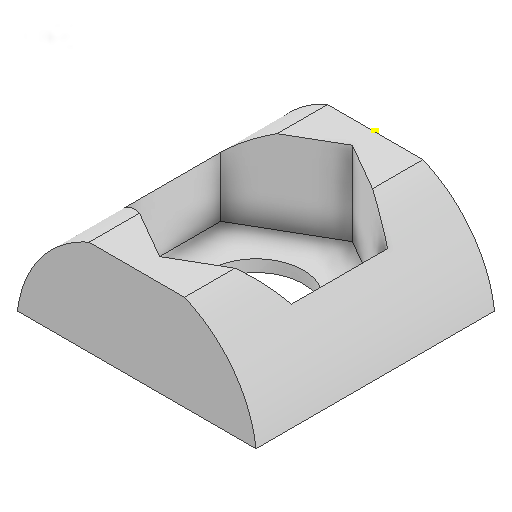
# Autodesk Inventor part: RailNut
Saved by Autodesk Inventor 2025.1 (Build 291241000, 241)
## iProperties
Created: 2025-03-12
Part Number: RailNut
Material: Generic
Document SubType Name: Modeling
Designer: rolan
Density: 1 g/cm^3
Appearance: Default
Author: rolan
Autodesk Inventor part; units mm, degrees
ref_plane "YZ Plane" through (0, 0, 0) normal (1, 0, 0) x (0, 1, 0)
ref_plane "XZ Plane" through (0, 0, 0) normal (0, 1, 0) x (-1, 0, 0)
ref_plane "XY Plane" through (0, 0, 0) normal (0, 0, 1) x (1, 0, 0)
sketch "Sketch1" plane through (0, 0, 0) normal (0, 0, 1) x (1, 0, 0)
  line L0 (-5, 0) -> (5, 0)
  line L1 (0, 0) -> (0, 4) construction
  line L2 (-2, 4) -> (2, 4)
  arc A0 (-2, 4) -> (-5, 0) centre (-0.0359, -0.5981) ccw
  arc A1 (5, 0) -> (2, 4) centre (0.0359, -0.5981) ccw
  dimension "d0" = 10
  dimension "d1" = 4
  dimension "d2" = 4
  dimension "d3" = 5
  dimension "d4" = 5
  constraints: 6 end point, 4 point on circle, 2 centre point, 2 horizontal, 2 midpoint, 1 vertical
  measures "d0" distance of L0.start L0.end
  measures "d1" distance of L1.start L1.end
  measures "d2" distance of L2.start L2.end
  measures "d3" radius of A0
  measures "d4" radius of A1
extrude "Extrusion1" add sketch "Sketch1" along normal blind 10
sketch "Sketch2" plane through (-2, 4, 0) normal (0, 1, 0) x (1, 0, 0)
  circle A0 centre (2, -5) radius 1.975
  line L0 (4, 0) -> (0, 0) projected
  line L1 (0, 0) -> (0, -10) projected
  point P0 (2, 0)
  point P1 (2, 0)
  dimension "d7" = 3.95
  dimension "d8" = 5
  dimension "d9" = 2
  constraints: 1 centre point, 1 midpoint
  measures "d7" diameter of A0
  measures "d8" distance of point (2, 0) A0.centre
  measures "d9" distance from line of L1 A0.centre
extrude "Extrusion2" cut sketch "Sketch2" against normal blind 10
sketch "Sketch3" plane through (-2, 4, 0) normal (0, 1, 0) x (1, 0, 0)
  point P0 (2, 0)
sketch "Sketch5" plane through (-2, 4, 0) normal (0, 1, 0) x (1, 0, 0)
  circle A0 centre (2, -5) radius 1.975 projected
  line L0 (2, -0.9585) -> (5.5, -2.9793)
  line L1 (5.5, -2.9793) -> (5.5, -7.0207)
  line L2 (5.5, -7.0207) -> (2, -9.0415)
  line L3 (2, -9.0415) -> (-1.5, -7.0207)
  line L4 (-1.5, -7.0207) -> (-1.5, -2.9793)
  line L5 (-1.5, -2.9793) -> (2, -0.9585)
  point P0 (2, 0)
  point P1 (5.5, -5)
  dimension "d15" = 3.5
  constraints: 12 end point, 1 coincident, 1 midpoint, 13 other
  measures "d15" distance of point (5.5, -5) point (2, -5)
extrude "Extrusion4" cut sketch "Sketch5" against normal blind 3.5
body "Solid1"
